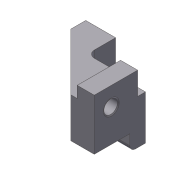
# Autodesk Inventor part: FOX-ME-121-05
Saved by Autodesk Inventor 2014 SP1 (Build 180222100, 222)
## iProperties
Created: 2011-09-07
Part Number: FOX-ME-121-05
Document SubType Name: Modeling
Designer: Robert Davis
Density: 2.71 g/cm^3
Material: Aluminum-6061
Mass: 4.06263 g
Surface Area: 12.1744 cm^2
Volume: 1.49912 cm^3
Description: RAIL END, -Z W/SWITCH
Appearance: Aluminum - Flat
Author: Robert Davis
Autodesk Inventor part; units mm, degrees
ref_plane "YZ Plane" through (0, 0, 0) normal (1, 0, 0) x (0, 1, 0)
ref_plane "XZ Plane" through (0, 0, 0) normal (0, 1, 0) x (-1, 0, 0)
ref_plane "XY Plane" through (0, 0, 0) normal (0, 0, 1) x (1, 0, 0)
sketch "Sketch1" plane through (0, 0, 0) normal (0, 0, 1) x (1, 0, 0)
  line L0 (-4.5, 4.25) -> (4.25, 4.25)
  line L1 (4.25, 4.25) -> (4.25, -4.5)
  line L2 (4.25, -4.5) -> (-4.5, -4.5)
  line L3 (-4.5, -4.5) -> (-4.5, 4.25)
  point P0 (0, 0)
  dimension "d0" = 8.75
  dimension "d1" = 8.75
  dimension "d2" = 4.25
  dimension "d3" = 4.25
  constraints: 8 end point, 2 horizontal, 2 vertical
  measures "d0" distance of L0.start L0.end
  measures "d1" distance of L0.end L1.end
  measures "d2" distance from line of L0 point (0, 0)
  measures "d3" distance from line of L1 point (0, 0)
extrude "Extrusion1" add sketch "Sketch1" along normal blind 2.8
fillet "Fillet2" radius 1 3 edges at (4.25, 4.25, 1.4) (4.25, -0.125, 0) (-0.125, 4.25, 0)
sketch "Sketch10" plane through (0, 0, 2.8) normal (0, 0, 1) x (1, 0, 0)
  line L0 (4.25, 3.25) -> (4.25, -4.5) projected
  line L1 (-4.5, 4.25) -> (3.25, 4.25) projected
  line L2 (3.25, 3.25) -> (-17.75, 3.25)
  line L3 (-17.75, 3.25) -> (-17.75, -17.75)
  line L4 (-17.75, -17.75) -> (3.25, -17.75)
  line L5 (3.25, -17.75) -> (3.25, 3.25)
  point P0 (0, 0)
  dimension "d113" = 1
  dimension "d114" = 1
  dimension "d115" = 21
  dimension "d116" = 21
  constraints: 8 end point
  measures "d113" distance between parallel lines of L0 L5
  measures "d114" distance between parallel lines of L2 L1
  measures "d115" distance of L2.start L2.end
  measures "d116" distance of L4.end L2.start
extrude "Extrusion8" add sketch "Sketch10" along normal blind 9
hole "Hole11" [suppressed]
sketch "Sketch11" plane through (0, 0, 2.8) normal (0, 0, -1) x (-1, 0, 0)
  line L0 (17.75, -17.75) -> (-3.25, -17.75) projected
  line L1 (17.75, 3.25) -> (17.75, -17.75) projected
  line L2 (4.5, 3.25) -> (17.75, 3.25) projected
  line L3 (12.25, 3.25) -> (17.75, 3.25)
  line L4 (17.75, 3.25) -> (17.75, -17.75)
  line L5 (17.75, -17.75) -> (-3.25, -17.75)
  line L6 (-3.25, -17.75) -> (-3.25, -10.75)
  line L7 (-3.25, -10.75) -> (2.25, -10.75)
  line L8 (2.25, -10.75) -> (12.25, -0.75)
  line L9 (12.25, -0.75) -> (12.25, 3.25)
  point P0 (0, 0)
  dimension "d146" = 14
  dimension "d158" = 4
  dimension "d254" = 15.5
  dimension "d255" = 45
  constraints: 14 end point, 3 horizontal, 3 vertical, 1 perpendicular, 1 point on line
  measures "d146" distance between parallel lines of L7 L2
  measures "d158" distance of L8.end L3.start
  measures "d254" distance between parallel lines of L6 L9
  measures "d255" angle of L0 L8
extrude "Extrusion9" cut sketch "Sketch11" along normal through all both and the other way through all
hole "Hole12" [suppressed]
hole "Hole13" [suppressed]
chamfer "Chamfer3" [suppressed]
chamfer "Chamfer4" [suppressed]
sketch "Sketch18" plane through (0, 0, 0) normal (0, 0, -1) x (-1, 0, 0)
  line L0 (7, 5.953) -> (7, -1.75)
  line L1 (7, -1.75) -> (-6.3618, -1.75)
  line L2 (-3.25, 3.25) -> (4.5, 3.25) projected
  line L3 (-3.25, -4.5) -> (-3.25, 3.25) projected
  line L4 (7, 5.953) -> (-6.3618, 5.953)
  line L5 (-6.3618, 5.953) -> (-6.3618, -1.75)
  point P0 (0, 0)
  dimension "d226" = 2.703
  dimension "d227" = 3.1118
  dimension "d228" = 5
  dimension "d229" = 10.25
  constraints: 8 end point, 1 horizontal, 1 vertical
  measures "d226" distance between parallel lines of L4 L2
  measures "d227" distance between parallel lines of L5 L3
  measures "d228" distance between parallel lines of L1 L2
  measures "d229" distance between parallel lines of L0 L3
extrude "Extrusion12" cut sketch "Sketch18" against normal through all
hole "Hole16" at (-0.5, -1.75, 6.1) direction (0, -1, 0) diameter 1.1913 depth 4 tip angle 118
pattern_linear "Rectangular Pattern1" [suppressed]
chamfer "Chamfer7" [suppressed]
sketch "Sketch19" plane through (-4.5, -1.75, 0) normal (0, 1, 0) x (1, 0, 0)
  circle A0 centre (4, -6.1) radius 0.5956 projected
  circle A1 centre (0.0078, -6.35) radius 0.5956
  point P0 (4.5, 0)
  dimension "d230" = 0.25
  dimension "d231" = 4
  constraints: 1 centre point, 1 equal radius
  measures "d230" vertical distance of A0.centre A1.centre
  measures "d231" distance of A0.centre A1.centre
extrude "Extrusion13" cut sketch "Sketch19" against normal blind 4 contours A1
sketch "Sketch21" plane through (0, 0, 2.8) normal (0, 0, -1) x (-1, 0, 0)
  line L0 (7, 3.25) -> (7, -1.75) projected
  line L1 (7, -1.75) -> (4.5, -1.75) projected
  line L2 (-3.25, -10.75) -> (-3.25, -4.5) projected
  line L3 (-3.25, -10.75) -> (2.25, -10.75) projected
  line L4 (2.25, -10.75) -> (12.25, -0.75) projected
  line L5 (12.25, -0.75) -> (12.25, 3.25) projected
  line L6 (7, 3.25) -> (12.25, 3.25) projected
  line L7 (12.25, 4.25) -> (12.25, -0.75)
  line L8 (12.25, -0.75) -> (2.25, -10.75)
  line L9 (2.25, -10.75) -> (-4.25, -10.75)
  line L10 (-4.25, -10.75) -> (-4.25, -4.5)
  line L11 (-4.25, -4.5) -> (4.5, -4.5)
  line L12 (4.5, -4.5) -> (4.5, -1.75)
  line L13 (4.5, -1.75) -> (7, -1.75)
  line L14 (7, -1.75) -> (7, 4.25)
  line L15 (7, 4.25) -> (12.25, 4.25)
  line L16 (-3.25, -4.5) -> (4.5, -4.5) projected
  line L17 (4.5, -4.5) -> (4.5, -1.75) projected
  point P0 (0, 0)
  dimension "d236" = 1
  dimension "d237" = 1
  constraints: 18 end point, 7 collinear, 1 horizontal, 1 vertical
  measures "d236" distance between parallel lines of L10 L2
  measures "d237" distance between parallel lines of L15 L6
extrude "Extrusion14" [suppressed]
chamfer "Chamfer8" [suppressed]
sketch "Sketch23" plane through (0, 0, 0) normal (0, 0, -1) x (-1, 0, 0)
  line L0 (-4.25, 4.25) -> (20.75, 4.25)
  line L1 (-4.25, -20.75) -> (-4.25, 4.25)
  line L2 (-1.875, -20.75) -> (-1.875, 1.875)
  line L3 (-1.875, 1.875) -> (20.75, 1.875)
  line L4 (4.5, -4.5) -> (4.5, -1.75) projected
  line L5 (20.75, 1.875) -> (20.75, 4.25)
  line L6 (-1.875, -20.75) -> (-4.25, -20.75)
  point P0 (0, 0)
  dimension "d245" = 2.375
  dimension "d249" = 1.875
  dimension "d250" = 1.875
  dimension "d251" = 25
  dimension "d252" = 25
  constraints: 12 end point, 3 perpendicular, 1 horizontal, 1 parallel, 1 vertical
  measures "d245" distance between parallel lines of L0 L3
  measures "d249" distance from line of point (0, 0) L3
  measures "d250" distance from line of point (0, 0) L2
  measures "d251" distance of L0.start L0.end
  measures "d252" distance between parallel lines of L6 L0
extrude "Extrusion16" cut sketch "Sketch23" against normal through all
hole "Hole10" at (-9.768, 1.875, 7.317) direction (0, -1, 0) diameter 2.3876 depth 5 tip angle 118 countersink diameter 2.794 countersink angle 120
fillet "Fillet4" radius 1 2 edges at (-1.3125, -4.5, 0) (-4.5, -3.125, 0)
hole "Hole18" at (1.875, -7.75, 8.5) direction (-1, 0, 0) diameter 2.3876 depth 4.826 tip angle 118 countersink diameter 2.794 countersink angle 120
hole "Hole17" at (-0.9768, -7.795, 2.8) direction (0, 0, 1) diameter 2.3876 depth 3.9878 tip angle 118 countersink diameter 2.794 countersink angle 120
sketch "Sketch24" plane through (0, 0, 11.8) normal (0, 0, 1) x (1, 0, 0)
  line L0 (1.875, -10.75) -> (1.875, -1.75) projected
  line L1 (-7, 1.875) -> (1.875, 1.875)
  line L2 (1.875, 1.875) -> (1.875, -3.125)
  line L3 (1.875, -3.125) -> (-7, -3.125)
  line L4 (-7, 1.875) -> (-7, -3.125)
  line L5 (-7, 1.875) -> (-12.25, 1.875) projected
  point P0 (0, 0)
  dimension "d276" = 5
  constraints: 8 end point, 2 perpendicular, 2 point on line, 1 collinear, 1 horizontal, 1 parallel
  measures "d276" distance of L1.end L2.end
extrude "Extrusion17" cut sketch "Sketch24" against normal blind 4
sketch "Sketch25" plane through (0, 0, 11.8) normal (0, 0, 1) x (1, 0, 0)
  line L0 (-12.25, 1.875) -> (-12.25, -0.75) projected
  line L1 (-12.25, -0.75) -> (-2.25, -10.75) projected
  line L2 (-12.25, 1.875) -> (-6.5, 1.875)
  line L3 (-6.5, 1.875) -> (-6.5, -6.5)
  line L4 (-6.5, -6.5) -> (-12.25, -6.5)
  line L5 (-12.25, -6.5) -> (-12.25, 1.875)
  point P0 (0, 0)
  constraints: 8 end point, 2 parallel, 1 horizontal, 1 perpendicular, 1 point on line
extrude "Extrusion18" cut sketch "Sketch25" against normal blind 2 contours L2 L3 L1 L0
sketch "Sketch26" plane through (0, 0, 11.8) normal (0, 0, 1) x (1, 0, 0)
  line L0 (-6.5, -3.125) -> (-6.5, -6.5) projected
  line L1 (-6.5, -6.5) -> (-2.25, -10.75) projected
  line L2 (-2.25, -10.75) -> (1.875, -10.75) projected
  line L3 (1.875, -10.75) -> (1.875, -3.125) projected
  line L4 (-6.5, -3.125) -> (-1.125, -3.125)
  line L5 (-1.125, -3.125) -> (-1.125, -10.75)
  line L6 (-1.125, -10.75) -> (-6.5, -10.75)
  line L7 (-6.5, -10.75) -> (-6.5, -3.125)
  point P0 (0, 0)
  dimension "d281" = 3
  constraints: 8 end point, 2 parallel, 1 horizontal, 1 perpendicular, 1 point on line
  measures "d281" distance between parallel lines of L5 L3
extrude "Extrusion19" cut sketch "Sketch26" against normal up to surface (2 mm away) contours L4 L5 L2 L1 L0
fillet "Fillet5" radius 1.3 1 edges at (-7, -3.125, 8.8)
body "Solid1"
